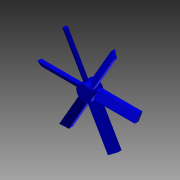
# Autodesk Inventor part: propeler
Saved by Autodesk Inventor 2012 (Build 160160000, 160)
## iProperties
Created: 2012-12-20
Part Number: propeler
Material: Default
Document SubType Name: Modeling
Designer: Irwan Haryanto
Density: 1 g/cm^3
Author: Irwan Haryanto
Autodesk Inventor part; units mm, degrees
ref_plane "XZ Plane" through (0, 0, 0) normal (0, 1, 0) x (-1, 0, 0)
ref_plane "XY Plane" through (0, 0, 0) normal (0, 0, 1) x (1, 0, 0)
sketch "Sketch1" plane through (0, 0, 0) normal (0, 0, 1) x (1, 0, 0)
  circle A0 centre (0, 0) radius 0.75
  circle A1 centre (0, 0) radius 4
  dimension "d0" = 1.5
  dimension "d1" = 8
  constraints: 2 centre point, 2 coincident
  measures "d0" diameter of A0
  measures "d1" diameter of A1
extrude "Extrusion1" add sketch "Sketch1" along normal blind 6 contours A0 | A1
extrude "Extrusion2" cut sketch "Sketch1" along normal blind 4 contours A0
ref_plane "Work Plane1" through (0, 0, 0) normal (1, 0, 0) x (0, 1, 0)
sketch "Sketch2" plane through (0, 0, 0) normal (1, 0, 0) x (0, 1, 0)
  line L0 (1.9777, 1) -> (-1.4864, 3)
  line L1 (1.9777, 1) -> (5.9777, 1) construction
  line L2 (1.9777, 1) -> (1.9777, 3)
  line L3 (1.9777, 3) -> (0.9602, 3.5874)
  line L4 (-4, 0) -> (4, 0) projected
  line L5 (0.9602, 3.5874) -> (-1.4864, 5)
  line L6 (-1.4864, 5) -> (-1.4864, 3)
  line L7 (-4, 6) -> (4, 6) projected
  point P0 (0, 0)
  dimension "d7" = 150
  dimension "d8" = 2
  dimension "d9" = 1
  dimension "d10" = 1
  constraints: 12 end point, 2 perpendicular, 1 collinear, 1 equal length, 1 horizontal, 1 parallel
  measures "d7" angle of L1 L0
  measures "d8" distance of L0.start L2.end
  measures "d9" distance from line of L0.start L4
  measures "d10" distance from line of L7 L5.end
extrude "Extrusion3" add sketch "Sketch2" along normal blind 25
sketch "Sketch3" plane through (0, 0, 0) normal (1, 0, 0) x (0, 1, 0)
  point P0 (0, 0)
pattern_circular "Circular Pattern1" count 6 over 360 about axis through (0, 0, 0) along (0, 0, 1) of "Extrusion3"
body "Solid1"
